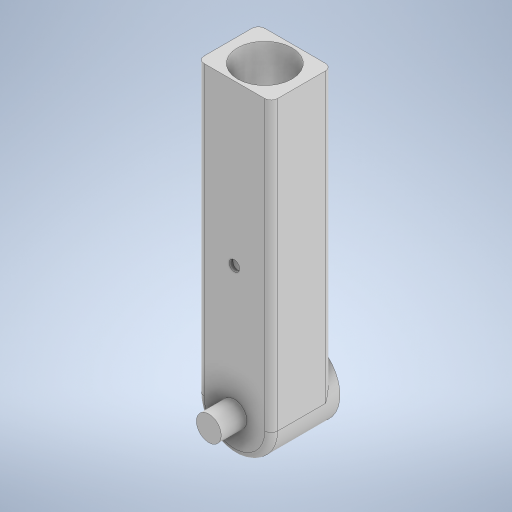
# Autodesk Inventor part: stick_mount
Saved by Autodesk Inventor 2023 (Build 270158000, 158)
## iProperties
Created: 2023-01-25
Part Number: stick_mount
Material: Generic
Document SubType Name: Modeling
Designer: Hunter
Density: 1 g/cm^3
Appearance: Default
Author: Hunter
Autodesk Inventor part; units mm, degrees
ref_plane "YZ Plane" through (0, 0, 0) normal (1, 0, 0) x (0, 1, 0)
ref_plane "XZ Plane" through (0, 0, 0) normal (0, 1, 0) x (-1, 0, 0)
ref_plane "XY Plane" through (0, 0, 0) normal (0, 0, 1) x (1, 0, 0)
sketch "Sketch1" plane through (0, 0, 0) normal (0, 0, 1) x (1, 0, 0)
  circle A0 centre (0, 0) radius 11.5
  dimension "d0" = 23
  constraints: 1 centre point, 1 coincident
  measures "d0" diameter of A0
extrude "Extrusion1" add sketch "Sketch1" along normal blind 26
sketch "Sketch2" plane through (0, 0, 0) normal (0, 1, 0) x (-1, 0, 0)
  line L0 (11.5, 0) -> (11.5, 26) projected
  line L1 (11.5, 26) -> (-11.5, 26) projected
  line L2 (11.5, 0) -> (-11.5, 0) projected
  line L3 (-11.5, 0) -> (-11.5, 26) projected
  line L4 (11.5, 0) -> (-11.5, 19) construction
  line L5 (-11.5, 0) -> (-11.5, 26) construction
  line L6 (-11.5, 0) -> (11.5, 19) construction
  line L7 (11.5, 0) -> (11.5, 26) construction
  line L8 (11.5, 19) -> (-11.5, 19) construction
  line L9 (11.5, 19) -> (-11.5, 19)
  line L10 (-11.5, 19) -> (-11.5, 0)
  line L11 (-11.5, 0) -> (11.5, 0)
  line L12 (11.5, 0) -> (11.5, 19)
  line L13 (11.5, 19) -> (-11.5, 0) construction
  line L14 (-11.5, 19) -> (11.5, 0) construction
  point P0 (0, 0)
  point P1 (11.5, 13)
  point P2 (0, 26)
  point P3 (0, 9.5)
  point P4 (0, 9.5)
  dimension "d15" = 7
  constraints: 18 end point, 6 midpoint, 3 point on line, 2 horizontal, 2 parallel, 1 perpendicular
  measures "d15" distance between parallel lines of L1 L8
extrude "Extrusion2" add sketch "Sketch2" along normal blind 90 contours L2 L3 L9 L0
sketch "Sketch3" plane through (0, 90, 7.5) normal (0, 1, 0) x (1, 0, 0)
  line L0 (-11.5, -11.5) -> (11.5, -11.5) construction
  line L1 (11.5, 7.5) -> (-11.5, 7.5) projected
  line L2 (11.5, -11.5) -> (11.5, 7.5) construction
  line L3 (-11.5, 7.5) -> (-11.5, -11.5) construction
  line L4 (-11.5, 7.5) -> (11.5, 7.5) construction
  circle A0 centre (0, -2) radius 8.5
  line L5 (11.5, -2) -> (-11.5, -2) construction
  line L6 (0, 7.5) -> (0, -11.5) construction
  dimension "d29" = 17
  constraints: 5 midpoint, 4 end point, 2 coincident, 1 centre point
  measures "d29" diameter of A0
extrude "Extrusion3" cut sketch "Sketch3" against normal blind 80
sketch "Sketch4" plane through (0, 0, 26) normal (0, 0, 1) x (1, 0, 0)
  circle A0 centre (0, 0) radius 3.9
  circle A1 centre (0, 0) radius 11.5
  dimension "d10" = 7.8
  dimension "d11" = 23
  constraints: 2 centre point, 2 coincident
  measures "d10" diameter of A0
  measures "d11" diameter of A1
extrude "Extrusion4" cut sketch "Sketch4" against normal blind 7
sketch "Sketch5" plane through (0, 0, 26) normal (0, 0, 1) x (1, 0, 0)
  circle A0 centre (0, 0) radius 3.9
  dimension "d18" = 7.8
  constraints: 1 centre point, 1 coincident
  measures "d18" diameter of A0
extrude "Extrusion5" add sketch "Sketch5" along normal blind 1
sketch "Sketch7" plane through (0, 0, 0) normal (0, 0, -1) x (-1, 0, 0)
  circle A0 centre (0, 0) radius 8 construction
  circle A1 centre (-2.6145, 7.5607) radius 1
  circle A2 centre (2.3849, 7.6363) radius 1
  circle A3 centre (7.531, 2.699) radius 1
  circle A4 centre (7.531, -2.699) radius 1
  circle A5 centre (2.3849, -7.6363) radius 1
  circle A6 centre (-2.6145, -7.5607) radius 1
  circle A7 centre (-7.4681, -2.8684) radius 1
  circle A8 centre (-7.4681, 2.8684) radius 1
  dimension "d31" = 16
  dimension "d32" = 15
  dimension "d33" = 15
  dimension "d34" = 5
  dimension "d35" = 5
  dimension "d36" = 2
  dimension "d37" = 2
  dimension "d38" = 2
  dimension "d39" = 2
  dimension "d40" = 2
  dimension "d41" = 2
  dimension "d42" = 2
  dimension "d43" = 2
  constraints: 9 coincident, 8 centre point, 10 other
  measures "d32" distance of point (7.531, 2.699) point (-7.468, 2.868)
  measures "d33" distance of point (7.531, -2.699) point (-7.468, -2.868)
  measures "d34" distance of point (2.385, 7.636) point (-2.615, 7.561)
  measures "d35" distance of point (2.385, -7.636) point (-2.615, -7.561)
  measures "d36" diameter of A1
  measures "d37" diameter of A2
  measures "d38" diameter of A3
  measures "d39" diameter of A4
  measures "d40" diameter of A5
  measures "d41" diameter of A6
  measures "d42" diameter of A7
  measures "d43" diameter of A8
extrude "Extrusion7" cut sketch "Sketch7" against normal blind 8
sketch "Sketch8" plane through (0, 0, 0) normal (0, 0, -1) x (-1, 0, 0)
  circle A0 centre (0, 0) radius 11.5
  circle A1 centre (0, 0) radius 10.5
  dimension "d46" = 23
  dimension "d47" = 21
  constraints: 2 centre point, 2 coincident
  measures "d46" diameter of A0
  measures "d47" diameter of A1
extrude "Extrusion8" add sketch "Sketch8" along normal blind 2.5
fillet "Fillet2" radius 2 5 edges at (0, -11.5, 19) (-11.5, 45, 19) (11.5, 45, 19) (11.5, 45, 0) (-11.5, 45, 0)
sketch "Sketch9" plane through (0, 0, 0) normal (0, 0, -1) x (-1, 0, 0)
  circle A0 centre (0, 40) radius 1.65
  line L0 (-9.5, 90) -> (9.5, 90) projected
  point P0 (0, 0)
  dimension "d51" = 3.3
  dimension "d52" = 50
  constraints: 1 centre point
  measures "d51" diameter of A0
  measures "d52" distance from line of L0 A0.centre
extrude "Extrusion9" cut sketch "Sketch9" against normal through all
body "Solid1"
